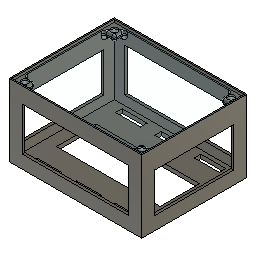
middle (Autodesk Fusion 360 design; units mm, degrees)
part number: 2026-02-02-18-42-25-237
Autodesk Fusion 360 part; units mm, degrees
sketch "Boceto1" plane through (0, 0, 0) normal (0, 0, 1) x (1, 0, 0)
  line L0 (0, 0) -> (101, 0)
  line L1 (101, 0) -> (101, 80)
  line L2 (101, 80) -> (0, 80)
  line L3 (0, 80) -> (0, 0)
  dimension "d1" = 101
  dimension "d2" = 80
  constraint horizontal L0
  constraint vertical L1
  constraint horizontal L2
  constraint vertical L3
  constraint coincident L0.start L3.end
  measures "d1" distance of L0.start L0.end
  measures "d2" distance of L0.start L2.end
extrude "Extruir1" add sketch "Boceto1" along normal blind 3
sketch "Boceto2" plane through (0, 0, 0) normal (0, 0, -1) x (1, 0, 0)
  line L0 (0, 0) -> (0, -80)
  line L1 (0, -80) -> (101, -80)
  line L2 (101, -80) -> (101, 0)
  line L3 (101, 0) -> (0, 0)
  line L4 (0, 0) -> (6, 0) construction
  line L5 (6, 0) -> (6, -6) construction
  line L6 (6, -6) -> (0, -6) construction
  line L7 (0, -6) -> (0, 0) construction
  constraint horizontal L4
  constraint vertical L5
  constraint horizontal L6
  constraint vertical L7
  constraint coincident L0.start L3.end
hole "Agujero1" at (6, 6, 0) direction (0, 0, 1) diameter 5.2 depth 1.2 tip angle 118
sketch "Boceto3" plane through (0, 0, 0) normal (0, 0, -1) x (1, 0, 0)
  circle A0 centre (6, -6) radius 2.6
  line L0 (0, 0) -> (0, -80)
  line L1 (0, -80) -> (101, -80)
  line L2 (101, -80) -> (101, 0)
  line L3 (101, 0) -> (0, 0)
  line L4 (0, -80) -> (6, -80)
  line L5 (6, -80) -> (6, -74)
  line L6 (6, -74) -> (0, -74)
  line L7 (0, -74) -> (0, -80)
  line L8 (101, -80) -> (95, -80)
  line L9 (95, -80) -> (95, -74)
  line L10 (95, -74) -> (101, -74)
  line L11 (101, -74) -> (101, -80)
  line L12 (101, 0) -> (95, 0)
  line L13 (95, 0) -> (95, -6)
  line L14 (95, -6) -> (101, -6)
  line L15 (101, -6) -> (101, 0)
  constraint horizontal L4
  constraint vertical L5
  constraint horizontal L6
  constraint vertical L7
  constraint coincident L0.end L1.start
  constraint horizontal L8
  constraint vertical L9
  constraint horizontal L10
  constraint vertical L11
  constraint coincident L1.end L2.start
  constraint horizontal L12
  constraint vertical L13
  constraint horizontal L14
  constraint vertical L15
  constraint coincident L2.end L3.start
hole "Agujero2" at (95, 6, 0) at (95, 74, 0) at (6, 74, 0) direction (0, 0, 1) diameter 5.2 depth 1.2 tip angle 118
extrude "Extruir2" add 1 faces at (33.6667, 53.3333, 3) along direction (0, 0, 1) blind 50
sketch "Boceto4" plane through (0, 0, 53) normal (0, 0, 1) x (-1, 0, 0)
  line L0 (0, -80) -> (0, 0)
  line L1 (0, 0) -> (-101, 0)
  line L2 (-101, 0) -> (-101, -80)
  line L3 (-101, -80) -> (0, -80)
  line L4 (-2, -2) -> (-99, -2)
  line L5 (-99, -2) -> (-99, -78)
  line L6 (-99, -78) -> (-2, -78)
  line L7 (-2, -78) -> (-2, -2)
  constraint horizontal L4
  constraint vertical L5
  constraint horizontal L6
  constraint vertical L7
extrude "Extruir3" cut sketch "Boceto4" against normal blind 50 contours L4 L5 L6 L7
sketch "Boceto5" plane through (0, 0, 0) normal (0, -1, 0) x (1, 0, 0)
  line L0 (0, 0) -> (101, 0)
  line L1 (101, 0) -> (101, 53)
  line L2 (101, 53) -> (0, 53)
  line L3 (0, 53) -> (0, 0)
  line L4 (10, 10) -> (91, 10)
  line L5 (91, 10) -> (91, 43)
  line L6 (91, 43) -> (10, 43)
  line L7 (10, 43) -> (10, 10)
  constraint horizontal L4
  constraint vertical L5
  constraint horizontal L6
  constraint vertical L7
extrude "Extruir4" cut sketch "Boceto5" against normal blind 100 contours L4 L5 L6 L7
sketch "Boceto6" plane through (101, 0, 0) normal (1, 0, 0) x (0, 1, 0)
  line L0 (0, 0) -> (80, 0)
  line L1 (80, 0) -> (80, 53)
  line L2 (80, 53) -> (0, 53)
  line L3 (0, 53) -> (0, 0)
  line L4 (10, 40) -> (70, 40)
  line L5 (70, 40) -> (70, 10)
  line L6 (70, 10) -> (10, 10)
  line L7 (10, 10) -> (10, 40)
  constraint horizontal L4
  constraint vertical L5
  constraint horizontal L6
  constraint vertical L7
extrude "Extruir5" cut sketch "Boceto6" against normal blind 1000 contours L4 L5 L6 L7
sketch "Boceto7" plane through (0, 0, 3) normal (0, 0, 1) x (-1, 0, 0)
  line L0 (-2, -78) -> (-2, -2)
  line L1 (-2, -2) -> (-99, -2)
  line L2 (-99, -2) -> (-99, -78)
  line L3 (-99, -78) -> (-2, -78)
  line L4 (-10, -75) -> (-30, -75)
  line L5 (-30, -75) -> (-30, -70)
  line L6 (-30, -70) -> (-10, -70)
  line L7 (-10, -70) -> (-10, -75)
  line L8 (-40, -75) -> (-60, -75)
  line L9 (-60, -75) -> (-60, -70)
  line L10 (-60, -70) -> (-40, -70)
  line L11 (-40, -70) -> (-40, -75)
  line L12 (-70, -75) -> (-90, -75)
  line L13 (-90, -75) -> (-90, -70)
  line L14 (-90, -70) -> (-70, -70)
  line L15 (-70, -70) -> (-70, -75)
  line L16 (-10, -5) -> (-30, -5)
  line L17 (-30, -5) -> (-30, -10)
  line L18 (-30, -10) -> (-10, -10)
  line L19 (-10, -10) -> (-10, -5)
  line L20 (-40, -10) -> (-60, -10)
  line L21 (-60, -10) -> (-60, -5)
  line L22 (-60, -5) -> (-40, -5)
  line L23 (-40, -5) -> (-40, -10)
  line L24 (-70, -10) -> (-90, -10)
  line L25 (-90, -10) -> (-90, -5)
  line L26 (-90, -5) -> (-70, -5)
  line L27 (-70, -5) -> (-70, -10)
  constraint horizontal L4
  constraint vertical L5
  constraint horizontal L6
  constraint vertical L7
  constraint horizontal L8
  constraint vertical L9
  constraint horizontal L10
  constraint vertical L11
  constraint horizontal L12
  constraint vertical L13
  constraint horizontal L14
  constraint vertical L15
  constraint horizontal L16
  constraint vertical L17
  constraint horizontal L18
  constraint vertical L19
  constraint horizontal L20
  constraint vertical L21
  constraint horizontal L22
  constraint vertical L23
  constraint horizontal L24
  constraint vertical L25
  constraint horizontal L26
  constraint vertical L27
extrude "Extruir6" cut sketch "Boceto7" against normal blind 100 contours L4 L5 L6 L7 | L8 L9 L10 L11 | L12 L13 L14 L15 | L16 L17 L18 L19 | L20 L21 L22 L23 | L24 L25 L26 L27
sketch "Boceto8" plane through (0, 0, 3) normal (0, 0, 1) x (-1, 0, 0)
  line L0 (-30, -75) -> (-30, -70)
  line L1 (-30, -70) -> (-10, -70)
  line L2 (-10, -70) -> (-10, -75)
  line L3 (-10, -75) -> (-30, -75)
  line L4 (-90, -10) -> (-90, -5)
  line L5 (-90, -5) -> (-70, -5)
  line L6 (-70, -5) -> (-70, -10)
  line L7 (-70, -10) -> (-90, -10)
  line L8 (-60, -75) -> (-60, -70)
  line L9 (-60, -70) -> (-40, -70)
  line L10 (-40, -70) -> (-40, -75)
  line L11 (-40, -75) -> (-60, -75)
  line L12 (-30, -5) -> (-10, -5)
  line L13 (-10, -5) -> (-10, -10)
  line L14 (-10, -10) -> (-30, -10)
  line L15 (-30, -10) -> (-30, -5)
  line L16 (-60, -10) -> (-60, -5)
  line L17 (-60, -5) -> (-40, -5)
  line L18 (-40, -5) -> (-40, -10)
  line L19 (-40, -10) -> (-60, -10)
  line L20 (-90, -75) -> (-90, -70)
  line L21 (-90, -70) -> (-70, -70)
  line L22 (-70, -70) -> (-70, -75)
  line L23 (-70, -75) -> (-90, -75)
  line L24 (-2, -78) -> (-2, -2)
  line L25 (-2, -2) -> (-99, -2)
  line L26 (-99, -2) -> (-99, -78)
  line L27 (-99, -78) -> (-2, -78)
  line L28 (-10, -55) -> (-90, -55)
  line L29 (-90, -55) -> (-90, -25)
  line L30 (-90, -25) -> (-10, -25)
  line L31 (-10, -25) -> (-10, -55)
  constraint horizontal L28
  constraint vertical L29
  constraint horizontal L30
  constraint vertical L31
extrude "Extruir7" cut sketch "Boceto8" against normal blind 100 contours L28 L29 L30 L31
sketch "Boceto9" plane through (0, 0, 53) normal (0, 0, 1) x (-1, 0, 0)
  line L0 (-99, -2) -> (-2, -2)
  line L1 (-2, -2) -> (-2, -78)
  line L2 (-2, -78) -> (-99, -78)
  line L3 (-99, -78) -> (-99, -2)
  line L4 (0, -80) -> (0, 0)
  line L5 (0, 0) -> (-101, 0)
  line L6 (-101, 0) -> (-101, -80)
  line L7 (-101, -80) -> (0, -80)
  line L8 (-99, -2) -> (-91, -2)
  line L9 (-91, -2) -> (-91, -10)
  line L10 (-91, -10) -> (-99, -10)
  line L11 (-99, -10) -> (-99, -2)
  constraint horizontal L8
  constraint vertical L9
  constraint horizontal L10
  constraint vertical L11
  constraint coincident L0.start L3.end
extrude "Extruir8" add sketch "Boceto9" against normal blind 5 contours L0 L3 L8 L9 L10 L11
ref_plane "PlanoDeObra1" through (50.5, 40, 26.5) normal (-1, 0, 0) x (0, -1, 0)
ref_plane "PlanoDeObra2" through (50.5, 40, 26.5) normal (0, -1, 0) x (1, 0, 0)
sketch "Boceto10" plane through (0, 0, 53) normal (0, 0, 1) x (-1, 0, 0)
  line L0 (-91, -2) -> (-2, -2)
  line L1 (-2, -2) -> (-2, -78)
  line L2 (-2, -78) -> (-99, -78)
  line L3 (-99, -78) -> (-99, -10)
  line L4 (-99, -10) -> (-91, -10)
  line L5 (-91, -10) -> (-91, -2)
  line L6 (0, -80) -> (0, 0)
  line L7 (0, 0) -> (-101, 0)
  line L8 (-101, 0) -> (-101, -80)
  line L9 (-101, -80) -> (0, -80)
  line L10 (-101, -6) -> (-95, -6) construction
  constraint coincident L8 L10.start
  constraint perpendicular L8 L10
hole "Agujero3" at (95, 6, 53) direction (0, 0, -1) diameter 5.2 depth 1.2 tip angle 118
fillet "Empalme1" radius 2 1 edges at (91, 2, 50.5) 3 faces at (96.3333, 4.6667, 48) (93.6667, 10, 49.6667) (91, 4.6667, 49.6667)
mirror "Simetría1" about plane through (50.5, 40, 26.5) normal (-1, 0, 0) of bodies 1 merged
mirror "Simetría2" about plane through (50.5, 40, 26.5) normal (0, -1, 0) of bodies 1 merged
sketch "Boceto11" plane through (0, 0, 53) normal (0, 0, 1) x (-1, 0, 0)
  line L0 (0, -80) -> (0, 0)
  line L1 (0, 0) -> (-101, 0)
  line L2 (-101, 0) -> (-101, -80)
  line L3 (-101, -80) -> (0, -80)
  line L4 (-2, -11.4641) -> (-2, -68.5359)
  spline S0 degree 3 poles (-4, -72) (-3.7229, -71.7229) (-3.4173, -71.4184) (-2.8579, -70.7703) (-2.6065, -70.4245) (-2.2999, -69.855) (-2.1892, -69.5981) (-2.0389, -69.0661) (-2, -68.7908) (-2, -68.5359) knots 0 0 0 0 0.117563 0.117563 0.235126 0.235126 0.311589 0.311589 0.388052 0.388052 0.388052 0.388052
  line L5 (-4, -72) -> (-4.3387, -72)
  arc A0 (-8, -75.6613) -> (-4.3387, -72) centre (-6, -74) ccw
  line L6 (-8, -75.6613) -> (-8, -76)
  spline S1 degree 3 poles (-11.4641, -78) (-11.2092, -78) (-10.9339, -77.9611) (-10.4019, -77.8108) (-10.145, -77.7001) (-9.5755, -77.3935) (-9.2297, -77.1421) (-8.5815, -76.5827) (-8.2771, -76.2771) (-8, -76) knots 1.011064 1.011064 1.011064 1.011064 1.087528 1.087528 1.163991 1.163991 1.281554 1.281554 1.399117 1.399117 1.399117 1.399117
  line L7 (-11.4641, -78) -> (-89.5359, -78)
  spline S2 degree 3 poles (-89.5359, -78) (-89.7908, -78) (-90.0661, -77.9611) (-90.5981, -77.8108) (-90.855, -77.7001) (-91.4245, -77.3935) (-91.7703, -77.1421) (-92.4185, -76.5827) (-92.7229, -76.2771) (-93, -76) knots 1.011064 1.011064 1.011064 1.011064 1.087528 1.087528 1.163991 1.163991 1.281554 1.281554 1.399117 1.399117 1.399117 1.399117
  line L8 (-93, -76) -> (-93, -75.6613)
  arc A1 (-96.6613, -72) -> (-93, -75.6613) centre (-95, -74) ccw
  line L9 (-96.6613, -72) -> (-97, -72)
  spline S3 degree 3 poles (-97, -72) (-97.2771, -71.7229) (-97.5827, -71.4184) (-98.1421, -70.7703) (-98.3935, -70.4245) (-98.7001, -69.855) (-98.8108, -69.5981) (-98.9611, -69.0661) (-99, -68.7908) (-99, -68.5359) knots 0 0 0 0 0.117563 0.117563 0.235126 0.235126 0.311589 0.311589 0.388052 0.388052 0.388052 0.388052
  line L10 (-99, -68.5359) -> (-99, -11.4641)
  spline S4 degree 3 poles (-97, -8) (-97.2771, -8.2771) (-97.5827, -8.5816) (-98.1421, -9.2297) (-98.3935, -9.5755) (-98.7001, -10.145) (-98.8108, -10.4019) (-98.9611, -10.9339) (-99, -11.2092) (-99, -11.4641) knots 0 0 0 0 0.117563 0.117563 0.235126 0.235126 0.311589 0.311589 0.388052 0.388052 0.388052 0.388052
  line L11 (-97, -8) -> (-96.6613, -8)
  arc A2 (-93, -4.3387) -> (-96.6613, -8) centre (-95, -6) ccw
  line L12 (-93, -4.3387) -> (-93, -4)
  spline S5 degree 3 poles (-89.5359, -2) (-89.7908, -2) (-90.0661, -2.0389) (-90.5981, -2.1892) (-90.855, -2.2999) (-91.4245, -2.6065) (-91.7703, -2.8579) (-92.4185, -3.4173) (-92.7229, -3.7229) (-93, -4) knots 1.011064 1.011064 1.011064 1.011064 1.087528 1.087528 1.163991 1.163991 1.281554 1.281554 1.399117 1.399117 1.399117 1.399117
  line L13 (-89.5359, -2) -> (-11.4641, -2)
  spline S6 degree 3 poles (-11.4641, -2) (-11.2092, -2) (-10.9339, -2.0389) (-10.4019, -2.1892) (-10.145, -2.2999) (-9.5755, -2.6065) (-9.2297, -2.8579) (-8.5815, -3.4173) (-8.2771, -3.7229) (-8, -4) knots 1.011064 1.011064 1.011064 1.011064 1.087528 1.087528 1.163991 1.163991 1.281554 1.281554 1.399117 1.399117 1.399117 1.399117
  line L14 (-8, -4) -> (-8, -4.3387)
  arc A3 (-4.3387, -8) -> (-8, -4.3387) centre (-6, -6) ccw
  line L15 (-4.3387, -8) -> (-4, -8)
  spline S7 degree 3 poles (-4, -8) (-3.7229, -8.2771) (-3.4173, -8.5816) (-2.8579, -9.2297) (-2.6065, -9.5755) (-2.2999, -10.145) (-2.1892, -10.4019) (-2.0389, -10.9339) (-2, -11.2092) (-2, -11.4641) knots 0 0 0 0 0.117563 0.117563 0.235126 0.235126 0.311589 0.311589 0.388052 0.388052 0.388052 0.388052
  line L16 (0, 0) -> (-101, 0)
  line L17 (-101, 0) -> (-101, -80)
  line L18 (-101, -80) -> (0, -80)
  line L19 (0, -80) -> (0, 0)
  line L20 (-1, -1) -> (-100, -1)
  line L21 (-100, -1) -> (-100, -79)
  line L22 (-100, -79) -> (-1, -79)
  line L23 (-1, -79) -> (-1, -1)
  constraint horizontal L16
  constraint vertical L17
  constraint horizontal L18
  constraint vertical L19
  constraint coincident L2.end L3.start
  constraint coincident L0.end L1.start
  constraint horizontal L20
  constraint vertical L21
  constraint horizontal L22
  constraint vertical L23
extrude "Extruir9" add sketch "Boceto11" along normal blind 2 contours L0 L1 L2 L3 L16 L17 L18 L19
sketch "Boceto12" plane through (0, 0, 53) normal (0, 0, 1) x (-1, 0, 0)
  line L0 (-1, -1) -> (-100, -1)
  line L1 (-100, -1) -> (-100, -79)
  line L2 (-100, -79) -> (-1, -79)
  line L3 (-1, -79) -> (-1, -1)
  line L4 (-2, -11.4641) -> (-2, -68.5359)
  spline S0 degree 3 poles (-4, -72) (-3.7229, -71.7229) (-3.4173, -71.4184) (-2.8579, -70.7703) (-2.6065, -70.4245) (-2.2999, -69.855) (-2.1892, -69.5981) (-2.0389, -69.0661) (-2, -68.7908) (-2, -68.5359) knots 0 0 0 0 0.117563 0.117563 0.235126 0.235126 0.311589 0.311589 0.388052 0.388052 0.388052 0.388052
  line L5 (-4, -72) -> (-4.3387, -72)
  arc A0 (-8, -75.6613) -> (-4.3387, -72) centre (-6, -74) ccw
  line L6 (-8, -75.6613) -> (-8, -76)
  spline S1 degree 3 poles (-11.4641, -78) (-11.2092, -78) (-10.9339, -77.9611) (-10.4019, -77.8108) (-10.145, -77.7001) (-9.5755, -77.3935) (-9.2297, -77.1421) (-8.5815, -76.5827) (-8.2771, -76.2771) (-8, -76) knots 1.011064 1.011064 1.011064 1.011064 1.087528 1.087528 1.163991 1.163991 1.281554 1.281554 1.399117 1.399117 1.399117 1.399117
  line L7 (-11.4641, -78) -> (-89.5359, -78)
  spline S2 degree 3 poles (-89.5359, -78) (-89.7908, -78) (-90.0661, -77.9611) (-90.5981, -77.8108) (-90.855, -77.7001) (-91.4245, -77.3935) (-91.7703, -77.1421) (-92.4185, -76.5827) (-92.7229, -76.2771) (-93, -76) knots 1.011064 1.011064 1.011064 1.011064 1.087528 1.087528 1.163991 1.163991 1.281554 1.281554 1.399117 1.399117 1.399117 1.399117
  line L8 (-93, -76) -> (-93, -75.6613)
  arc A1 (-96.6613, -72) -> (-93, -75.6613) centre (-95, -74) ccw
  line L9 (-96.6613, -72) -> (-97, -72)
  spline S3 degree 3 poles (-97, -72) (-97.2771, -71.7229) (-97.5827, -71.4184) (-98.1421, -70.7703) (-98.3935, -70.4245) (-98.7001, -69.855) (-98.8108, -69.5981) (-98.9611, -69.0661) (-99, -68.7908) (-99, -68.5359) knots 0 0 0 0 0.117563 0.117563 0.235126 0.235126 0.311589 0.311589 0.388052 0.388052 0.388052 0.388052
  line L10 (-99, -68.5359) -> (-99, -11.4641)
  spline S4 degree 3 poles (-97, -8) (-97.2771, -8.2771) (-97.5827, -8.5816) (-98.1421, -9.2297) (-98.3935, -9.5755) (-98.7001, -10.145) (-98.8108, -10.4019) (-98.9611, -10.9339) (-99, -11.2092) (-99, -11.4641) knots 0 0 0 0 0.117563 0.117563 0.235126 0.235126 0.311589 0.311589 0.388052 0.388052 0.388052 0.388052
  line L11 (-97, -8) -> (-96.6613, -8)
  arc A2 (-93, -4.3387) -> (-96.6613, -8) centre (-95, -6) ccw
  line L12 (-93, -4.3387) -> (-93, -4)
  spline S5 degree 3 poles (-89.5359, -2) (-89.7908, -2) (-90.0661, -2.0389) (-90.5981, -2.1892) (-90.855, -2.2999) (-91.4245, -2.6065) (-91.7703, -2.8579) (-92.4185, -3.4173) (-92.7229, -3.7229) (-93, -4) knots 1.011064 1.011064 1.011064 1.011064 1.087528 1.087528 1.163991 1.163991 1.281554 1.281554 1.399117 1.399117 1.399117 1.399117
  line L13 (-89.5359, -2) -> (-11.4641, -2)
  spline S6 degree 3 poles (-11.4641, -2) (-11.2092, -2) (-10.9339, -2.0389) (-10.4019, -2.1892) (-10.145, -2.2999) (-9.5755, -2.6065) (-9.2297, -2.8579) (-8.5815, -3.4173) (-8.2771, -3.7229) (-8, -4) knots 1.011064 1.011064 1.011064 1.011064 1.087528 1.087528 1.163991 1.163991 1.281554 1.281554 1.399117 1.399117 1.399117 1.399117
  line L14 (-8, -4) -> (-8, -4.3387)
  arc A3 (-4.3387, -8) -> (-8, -4.3387) centre (-6, -6) ccw
  line L15 (-4.3387, -8) -> (-4, -8)
  spline S7 degree 3 poles (-4, -8) (-3.7229, -8.2771) (-3.4173, -8.5816) (-2.8579, -9.2297) (-2.6065, -9.5755) (-2.2999, -10.145) (-2.1892, -10.4019) (-2.0389, -10.9339) (-2, -11.2092) (-2, -11.4641) knots 0 0 0 0 0.117563 0.117563 0.235126 0.235126 0.311589 0.311589 0.388052 0.388052 0.388052 0.388052
equation "d25 = ( -101 / 2 ) * 1 mm"
